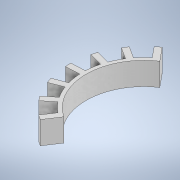
# Autodesk Inventor part: pneunet_approximate_test_first_bend
Saved by Autodesk Inventor 2021 (Build 250183000, 183)
## iProperties
Created: 2021-03-25
Part Number: pneunet_approximate_test_first_bend
Material: Generic
Document SubType Name: Modeling
Designer: Charlie
Density: 1 g/cm^3
Appearance: Default
Author: Charlie
Autodesk Inventor part; units mm, degrees
ref_plane "YZ Plane" through (0, 0, 0) normal (1, 0, 0) x (0, 1, 0)
ref_plane "XZ Plane" through (0, 0, 0) normal (0, 1, 0) x (-1, 0, 0)
ref_plane "XY Plane" through (0, 0, 0) normal (0, 0, 1) x (1, 0, 0)
sketch "Sketch1" plane through (0, 0, 0) normal (0, 1, 0) x (-1, 0, 0)
  line L0 (-34.333, 34.6818) -> (-49.333, 34.6818) construction
  line L1 (-34.333, -45.5191) -> (-34.333, 34.6818) construction
  line L2 (-34.333, 34.6818) -> (-49.333, -49.911) construction
  line L3 (-34.333, 34.6818) -> (-34.333, 29.6818) construction
  line L4 (-34.333, 19.6818) -> (-46.333, 19.6818) construction
  line L5 (-46.333, 19.6818) -> (-46.333, 29.6818) construction
  line L6 (-46.333, 29.6818) -> (-34.333, 29.6818) construction
  line L7 (-34.333, 3.6818) -> (-46.333, 3.6818) construction
  line L8 (-46.333, 3.6818) -> (-46.333, 13.6818) construction
  line L9 (-46.333, 13.6818) -> (-34.333, 13.6818) construction
  line L10 (-34.333, -12.3182) -> (-46.333, -12.3182) construction
  line L11 (-46.333, -12.3182) -> (-46.333, -2.3182) construction
  line L12 (-46.333, -2.3182) -> (-34.333, -2.3182) construction
  line L13 (-34.333, -28.3182) -> (-46.333, -28.3182) construction
  line L14 (-46.333, -28.3182) -> (-46.333, -18.3182) construction
  line L15 (-46.333, -18.3182) -> (-34.333, -18.3182) construction
  line L16 (-34.333, -44.3182) -> (-46.333, -44.3182) construction
  line L17 (-46.333, -44.3182) -> (-46.333, -34.3182) construction
  line L18 (-46.333, -34.3182) -> (-34.333, -34.3182) construction
  line L19 (-34.333, -60.3182) -> (-46.333, -60.3182) construction
  line L20 (-46.333, -60.3182) -> (-46.333, -50.3182) construction
  line L21 (-46.333, -50.3182) -> (-34.333, -50.3182) construction
  line L22 (-34.333, 19.6818) -> (-34.333, 13.6818) construction
  line L23 (-34.333, 3.6818) -> (-34.333, -2.3182) construction
  line L24 (-34.333, -12.3182) -> (-34.333, -18.3182) construction
  line L25 (-34.333, -28.3182) -> (-34.333, -34.3182) construction
  arc A0 (-7.5, -42.2964) -> (-7.5, 42.2964) centre (-35.5563, 0) ccw
  line L26 (-49.333, 34.6818) -> (-49.333, -65.3182) construction
  line L27 (-49.333, -65.3182) -> (-34.333, -65.3182) construction
  line L28 (-34.333, -65.3182) -> (-34.333, -60.3182) construction
  line L29 (0.7921, 54.796) -> (-7.5, 42.2964)
  line L30 (0.7921, 54.796) -> (4.9587, 52.032)
  line L31 (-1.8037, 41.8383) -> (4.9587, 52.032)
  line L32 (9.3874, 29.4913) -> (18.9468, 37.1243)
  line L33 (15.8269, 41.0315) -> (18.9468, 37.1243)
  line L34 (15.8269, 41.0315) -> (4.1052, 31.6719)
  line L35 (16.2597, 14.3103) -> (27.6972, 18.649)
  line L36 (25.9239, 23.3239) -> (27.6972, 18.649)
  line L37 (25.9239, 23.3239) -> (11.899, 18.0039)
  line L38 (18.1525, -2.2458) -> (30.3692, -1.6184)
  line L39 (30.1128, 3.375) -> (30.3692, -1.6184)
  line L40 (30.1128, 3.375) -> (15.1325, 2.6057)
  line L41 (14.8841, -18.5862) -> (26.706, -21.7303)
  line L42 (27.9911, -16.8982) -> (26.706, -21.7303)
  line L43 (27.9911, -16.8982) -> (13.495, -13.0429)
  line L44 (6.7685, -33.1405) -> (17.0595, -39.7539)
  line L45 (19.7626, -35.5476) -> (17.0595, -39.7539)
  line L46 (19.7626, -35.5476) -> (7.1437, -27.4381)
  line L47 (-5.4144, -44.51) -> (2.3568, -53.9573)
  line L48 (6.2182, -50.781) -> (2.3568, -53.9573)
  line L49 (6.2182, -50.781) -> (-3.3108, -39.1966)
  arc A1 (-5.4144, -44.51) -> (-5.8417, 44.7964) centre (-35.5563, 0) ccw
  line L50 (2.3568, -53.9573) -> (-7.329, -42.1825)
  point P0 (0, 0)
  point P1 (-34.333, -5.4186)
  point P2 (-1.405, -41.5135)
  point P3 (9.6675, -29.06)
  point P4 (16.3942, -13.814)
  point P5 (18.1286, 2.7595)
  point P6 (14.704, 19.0679)
  point P7 (6.4495, 33.5438)
  point P8 (-7.5, 42.2964)
  dimension "d4" = 5
  dimension "d5" = 10
  dimension "d6" = 12
  dimension "d9" = 16
  dimension "d14" = 10
  dimension "d19" = 100
  dimension "d20" = 3
  dimension "d25" = 5
  dimension "d28" = 107
  dimension "d30" = 17.833
  dimension "d31" = 50.7557
  constraints: 102 end point, 6 point on circle, 4 equal length, 3 perpendicular, 2 centre point, 2 point on line, 2 vertical, 1 horizontal, 1 midpoint, 78 other
  measures "d4" distance of L0.start L3.end
  measures "d5" distance of L3.end L4.start
  measures "d6" distance of L4.start L4.end
  measures "d9" distance of L4.start L7.start
  measures "d14" distance of L13.end L14.end
  measures "d19" distance of L0.end L26.end
  measures "d20" distance between parallel lines of L26 L20
  measures "d25" distance of L29.start L30.end
  measures "d30" angle of L40 L35
  measures "d31" radius of A0
extrude "Extrusion1" add sketch "Sketch1" along normal blind 20
body "Solid1"
